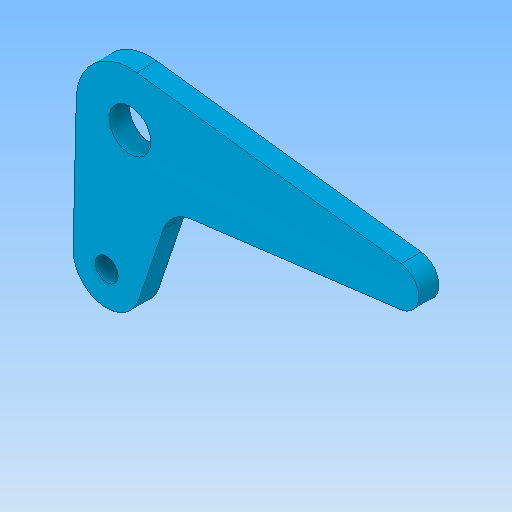
# Autodesk Inventor part: Pancake_Lever
Saved by Autodesk Inventor 2018.1 (Build 221171000, 171)
## iProperties
Created: 2019-02-11
Part Number: Pancake_Lever
Material: Nylon 6/6
Document SubType Name: Modeling
Designer: James
Density: 1.13 g/cm^3
Appearance: Sky Blue Medium
Mass: 2.43367 g
Surface Area: 19.5967 cm^2
Volume: 2.15369 cm^3
Author: James
Autodesk Inventor part; units mm, degrees
ref_plane "YZ Plane" through (0, 0, 0) normal (1, 0, 0) x (0, 1, 0)
ref_plane "XZ Plane" through (0, 0, 0) normal (0, 1, 0) x (-1, 0, 0)
ref_plane "XY Plane" through (0, 0, 0) normal (0, 0, 1) x (1, 0, 0)
sketch "Sketch1" plane through (0, 0, 0) normal (0, 0, 1) x (1, 0, 0)
  circle A0 centre (0, 0) radius 8
  line L0 (1, 7.9373) -> (40.375, 2.9765)
  line L1 (1, -7.9373) -> (40.375, -2.9765)
  line L2 (0, 0) -> (40, 0) construction
  circle A1 centre (40, 0) radius 3
  circle A2 centre (-3.473, -19.6962) radius 5
  line L3 (1.2651, -21.2932) -> (7.5809, -2.5552)
  line L4 (-8.4715, -19.5763) -> (-7.9977, 0.1917)
  line L5 (0, 0) -> (-3.473, -19.6962) construction
  dimension "d0" = 16
  dimension "d1" = 6
  dimension "d2" = 40
  dimension "d3" = 10
  dimension "d4" = 20
  dimension "d5" = 100
  constraints: 12 end point, 8 point on circle, 8 tangent, 3 centre point, 2 coincident, 1 horizontal
  measures "d0" diameter of A0
  measures "d1" diameter of A1
  measures "d2" distance of L2.end point (0, 0)
  measures "d3" diameter of A2
  measures "d4" distance of L2.start L5.end
  measures "d5" angle of L2 L5
extrude "Extrusion1" add sketch "Sketch1" along normal blind 3
fillet "Fillet1" radius 5 1 edges at (5.9783, -7.31, 1.5)
sketch "Sketch2" plane through (0, 0, 3) normal (0, 0, 1) x (1, 0, 0)
  point P0 (0, 0)
  point P1 (0, 0)
  constraints: 1 coincident
hole "Hole1" at (0, 0, 3) direction (0, 0, -1) diameter 6.2 end through all
sketch "Sketch3" plane through (0, 0, 3) normal (0, 0, 1) x (1, 0, 0)
  arc A0 (-8.4715, -19.5763) -> (1.2651, -21.2932) centre (-3.473, -19.6962) ccw projected
  point P0 (0, 0)
  constraints: 1 coincident
hole "Hole2" at (-3.473, -19.6962, 3) direction (0, 0, -1) diameter 3.4 end through all clearance for "Socket Head Cap Screw" size "M3" standard "Ansi Metric M Profile"
body "Solid1"
